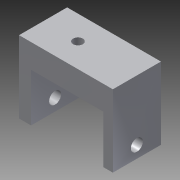
# Autodesk Inventor part: tiny clevis
Saved by Autodesk Inventor 2013 (Build 170138000, 138)
## iProperties
Created: 2013-02-05
Part Number: tiny clevis
Material: Aluminum 6061
Document SubType Name: Modeling
Designer: Arpan
Density: 1 g/cm^3
Author: Arpan
Autodesk Inventor part; units mm, degrees
ref_plane "YZ Plane" through (0, 0, 0) normal (1, 0, 0) x (0, 1, 0)
ref_plane "XZ Plane" through (0, 0, 0) normal (0, 1, 0) x (-1, 0, 0)
ref_plane "XY Plane" through (0, 0, 0) normal (0, 0, 1) x (1, 0, 0)
sketch "Sketch1" plane through (0, 0, 0) normal (0, 0, 1) x (1, 0, 0)
  line L0 (0, 0) -> (0, 12.7)
  line L1 (0, 12.7) -> (-19.05, 12.7)
  line L2 (-19.05, 12.7) -> (-19.05, 0)
  line L3 (-19.05, 0) -> (-22.225, 0)
  line L4 (-22.225, 0) -> (-22.225, 19.05)
  line L5 (-22.225, 19.05) -> (2.54, 19.05)
  line L6 (2.54, 19.05) -> (2.54, 0)
  line L7 (2.54, 0) -> (0, 0)
  dimension "d0" = 12.7
  dimension "d1" = 19.05
  dimension "d2" = 3.175
  dimension "d4" = 19.05
  dimension "d5" = 24.765
  constraints: 16 end point, 6 perpendicular, 1 parallel, 1 vertical
  measures "d0" distance of L0.start L0.end
  measures "d1" distance of L0.end L1.end
  measures "d2" distance of L2.end L3.end
  measures "d4" distance of L3.end L4.end
  measures "d5" distance of L4.end L5.end
extrude "Extrusion1" add sketch "Sketch1" along normal blind 12.7
sketch "Sketch2" plane through (-22.225, 19.05, 0) normal (0, 1, 0) x (1, 0, 0)
  line L0 (0, 0) -> (0, -12.7) projected
  line L1 (24.765, 0) -> (24.765, -12.7) projected
  line L2 (0, -6.35) -> (9.2075, -6.35)
  circle A0 centre (9.2075, -6.35) radius 1.2891
  point P0 (22.225, 0)
  dimension "d8" = 2.5781
  constraints: 2 end point, 1 centre point, 1 coincident, 1 midpoint, 1 perpendicular
  measures "d8" diameter of A0
extrude "Extrusion2" cut sketch "Sketch2" against normal blind 25.4
sketch "Sketch3" plane through (2.54, 0, 0) normal (1, 0, 0) x (0, 0, -1)
  line L0 (0, 0) -> (-12.7, 0) projected
  line L1 (-6.35, 0) -> (-6.35, 3.175)
  circle A0 centre (-6.35, 3.175) radius 1.5875
  dimension "d12" = 3.175
  dimension "d14" = 3.175
  constraints: 2 end point, 1 centre point, 1 coincident, 1 midpoint, 1 perpendicular
  measures "d12" distance of L1.start L1.end
  measures "d14" diameter of A0
extrude "Extrusion3" cut sketch "Sketch3" against normal blind 25.4
body "Solid1"
